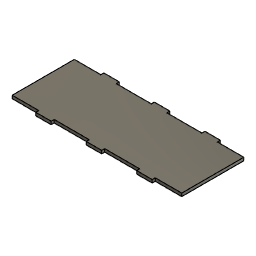
GBS 8200 Seitenteil v2 (Autodesk Fusion 360 design; units mm, degrees)
Autodesk Fusion 360 part; units mm, degrees
sketch "Skizze1" plane through (0, 0, 0) normal (0, 1, 0) x (1, 0, 0)
  line L0 (0, 0) -> (101, 0)
  line L1 (101, 0) -> (101, 40.6)
  line L2 (101, 40.6) -> (0, 40.6)
  line L3 (0, 40.6) -> (0, 0)
  line L4 (0, 0) -> (15.8, 0)
  line L5 (15.8, 0) -> (15.8, 1.8)
  line L6 (15.8, 1.8) -> (0, 1.8)
  line L7 (0, 1.8) -> (0, 0)
  line L8 (25, 0) -> (45.9, 0)
  line L9 (45.9, 0) -> (45.9, 1.8)
  line L10 (45.9, 1.8) -> (25, 1.8)
  line L11 (25, 1.8) -> (25, 0)
  line L12 (55.1, 0) -> (76, 0)
  line L13 (76, 0) -> (76, 1.8)
  line L14 (76, 1.8) -> (55.1, 1.8)
  line L15 (55.1, 1.8) -> (55.1, 0)
  line L16 (85.2, 0) -> (101, 0)
  line L17 (101, 0) -> (101, 1.8)
  line L18 (101, 1.8) -> (85.2, 1.8)
  line L19 (85.2, 1.8) -> (85.2, 0)
  line L20 (0, 40.6) -> (15.8, 40.6)
  line L21 (15.8, 40.6) -> (15.8, 38.8)
  line L22 (15.8, 38.8) -> (0, 38.8)
  line L23 (0, 38.8) -> (0, 40.6)
  line L24 (25, 40.6) -> (45.9, 40.6)
  line L25 (45.9, 40.6) -> (45.9, 38.8)
  line L26 (45.9, 38.8) -> (25, 38.8)
  line L27 (25, 38.8) -> (25, 40.6)
  line L28 (55.1, 40.6) -> (76, 40.6)
  line L29 (76, 40.6) -> (76, 38.8)
  line L30 (76, 38.8) -> (55.1, 38.8)
  line L31 (55.1, 38.8) -> (55.1, 40.6)
  line L32 (101, 40.6) -> (85.2, 40.6)
  line L33 (85.2, 40.6) -> (85.2, 38.8)
  line L34 (85.2, 38.8) -> (101, 38.8)
  line L35 (101, 38.8) -> (101, 40.6)
  dimension "d1" = 101
  dimension "d2" = 40.6
  dimension "d3" = 15.8
  dimension "d4" = 1.8
  dimension "d6" = 1.8
  dimension "d7" = 9.2
  dimension "d8" = 45.9
  dimension "d9" = 1.8
  dimension "d10" = 9.2
  dimension "d14" = 15.8
  dimension "d15" = 9.2
  dimension "d16" = 15.8
  dimension "d17" = 1.8
  dimension "d18" = 1.8
  dimension "d19" = 9.2
  dimension "d20" = 45.9
  dimension "d22" = 15.8
  dimension "d23" = 1.8
  dimension "d24" = 9.2
  dimension "d25" = 9.2
  constraint horizontal L0
  constraint vertical L1
  constraint horizontal L2
  constraint vertical L3
  constraint coincident L0.start L3.end
  constraint horizontal L4
  constraint vertical L5
  constraint horizontal L6
  constraint vertical L7
  constraint horizontal L8
  constraint vertical L9
  constraint horizontal L10
  constraint vertical L11
  constraint coincident L0 L8.start
  constraint horizontal L12
  constraint vertical L13
  constraint horizontal L14
  constraint vertical L15
  constraint coincident L0 L12.start
  constraint horizontal L16
  constraint vertical L17
  constraint horizontal L18
  constraint vertical L19
  constraint coincident L1 L17.end
  constraint coincident L0 L16.start
  constraint horizontal L20
  constraint vertical L21
  constraint horizontal L22
  constraint vertical L23
  constraint horizontal L24
  constraint vertical L25
  constraint horizontal L26
  constraint vertical L27
  constraint coincident L2 L24.start
  constraint horizontal L28
  constraint vertical L29
  constraint horizontal L30
  constraint vertical L31
  constraint coincident L2 L28.start
  constraint horizontal L32
  constraint vertical L33
  constraint horizontal L34
  constraint vertical L35
  measures "d1" distance of L0.start L0.end
  measures "d2" distance of L0.start L2.end
  measures "d3" distance of L0.start L4.end
  measures "d4" distance of L0.start L6.end
  measures "d6" distance of L8.start L10.end
  measures "d7" distance of L5 L11
  measures "d8" distance of L0.start L8.end
  measures "d9" distance of L12.start L14.end
  measures "d10" distance of L8.end L12.start
  measures "d14" distance of L17.end L18.end
  measures "d15" distance of L13.end L18.end
  measures "d16" distance of L2.end L20.end
  measures "d17" distance of L2.end L22.end
  measures "d18" distance of L24.start L26.end
  measures "d19" distance of L21.end L26.end
  measures "d20" distance of L22.end L25.end
  measures "d22" distance of L1.end L32.end
  measures "d23" distance of L1.end L34.end
  measures "d24" distance of L29.end L33.end
  measures "d25" distance of L25.end L30.end
extrude "Extrusion1" add sketch "Skizze1" along normal blind 1.8 contours L0 L1 L2 L3 L5 L6 L9 L10 L11 L13 L14 L15 L18 L19 L21 L22 L25 L26 L27 L29 L30 L31 L33 L34
